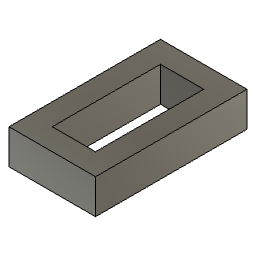
Spacer v2 (Autodesk Fusion 360 design; units mm, degrees)
Autodesk Fusion 360 part; units mm, degrees
sketch "Sketch1" plane through (0, 0, 0) normal (0, 0, 1) x (1, 0, 0)
  line L0 (10, -17.5) -> (-10, -17.5)
  line L1 (-10, -17.5) -> (-10, 17.5)
  line L2 (-10, 17.5) -> (10, 17.5)
  line L3 (10, 17.5) -> (10, -17.5)
  line L4 (10, -17.5) -> (-10, 17.5) construction
  line L5 (-10, -17.5) -> (10, 17.5) construction
  line L6 (5, -12.5) -> (-5, -12.5)
  line L7 (-5, -12.5) -> (-5, 12.5)
  line L8 (-5, 12.5) -> (5, 12.5)
  line L9 (5, 12.5) -> (5, -12.5)
  line L10 (5, -12.5) -> (-5, 12.5) construction
  line L11 (-5, -12.5) -> (5, 12.5) construction
  dimension "d1" = 35
  dimension "d2" = 25
  constraint horizontal L0
  constraint perpendicular L0 L1
  constraint parallel L0 L2
  constraint parallel L1 L3
  constraint coincident L4 origin
  constraint coincident L5 origin
  constraint horizontal L6
  constraint perpendicular L6 L7
  constraint parallel L6 L8
  constraint parallel L7 L9
  constraint coincident L10 origin
  constraint coincident L11 origin
  measures "d1" distance of L0.end L1.end
  measures "d2" distance of L6.end L7.end
extrude "Extrude1" add sketch "Sketch1" along normal blind 8
named bodies: "AS Spacer"
